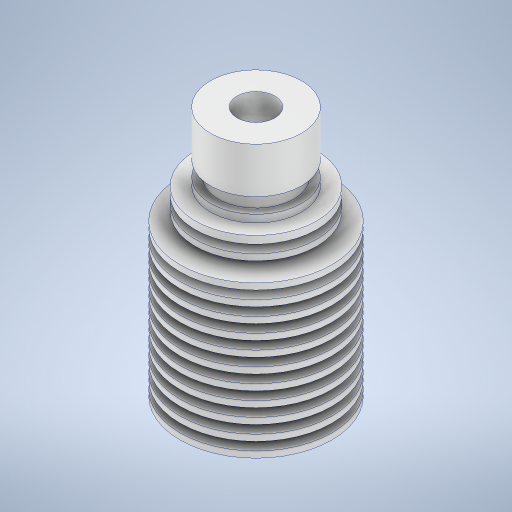
# Autodesk Inventor part: REVO-micro Heatsing body
Saved by Autodesk Inventor 2023.1 (Build 271208000, 208)
## iProperties
Created: 2022-11-20
Part Number: REVO-micro Heatsing body
Material: Aluminum 6061
Document SubType Name: Modeling
Designer: Frank
Density: 2.7 g/cm^3
Appearance: Aluminum - Flat
Mass: 12.3823 g
Surface Area: 79.4067 cm^2
Volume: 4.58604 cm^3
Author: Frank
Autodesk Inventor part; units mm, degrees
ref_plane "YZ Plane" through (0, 0, 0) normal (1, 0, 0) x (0, 1, 0)
ref_plane "XZ Plane" through (0, 0, 0) normal (0, 1, 0) x (-1, 0, 0)
ref_plane "XY Plane" through (0, 0, 0) normal (0, 0, 1) x (1, 0, 0)
sketch "Sketch1" plane through (0, 0, 0) normal (0, 0, 1) x (1, 0, 0)
  line L0 (0, 33) -> (0, -1)
  line L1 (0, -1) -> (3.75, -1) construction
  line L2 (3.75, -1) -> (3.75, 0)
  line L3 (3.75, 0) -> (10, 0)
  line L4 (10, 0) -> (10, 20)
  line L5 (10, 20) -> (8, 20)
  line L6 (8, 20) -> (8, 24)
  line L7 (8, 24) -> (6, 24)
  line L8 (6, 24) -> (6, 25)
  line L9 (6, 25) -> (5, 25)
  line L10 (5, 25) -> (5, 27)
  line L11 (5, 27) -> (6, 27)
  line L12 (6, 27) -> (6, 33)
  line L13 (6, 33) -> (0, 33)
  line L14 (10, 0) -> (0, 0) construction
  line L15 (6, 24) -> (6, 33) construction
  line L16 (2.5, 33) -> (2.5, 19)
  line L17 (2.5, 19) -> (1.55, 19)
  line L18 (1.55, 19) -> (1.55, 17)
  line L19 (1.55, 17) -> (2, 17)
  line L20 (10, 19.1818) -> (4.75, 19.1818)
  line L21 (4.75, 19.1818) -> (4.75, 18.0818)
  line L22 (4.75, 18.0818) -> (10, 18.0818)
  line L23 (10, 17.2636) -> (4.75, 17.2636)
  line L24 (4.75, 16.1636) -> (4.75, 17.2636)
  line L25 (4.75, 16.1636) -> (10, 16.1636)
  line L26 (10, 15.3455) -> (4.75, 15.3455)
  line L27 (4.75, 15.3455) -> (4.75, 14.2455)
  line L28 (4.75, 14.2455) -> (10, 14.2455)
  line L29 (10, 13.4273) -> (4.75, 13.4273)
  line L30 (4.75, 13.4273) -> (4.75, 12.3273)
  line L31 (4.75, 12.3273) -> (10, 12.3273)
  line L32 (10, 11.5091) -> (4.75, 11.5091)
  line L33 (4.75, 11.5091) -> (4.75, 10.4091)
  line L34 (4.75, 10.4091) -> (10, 10.4091)
  line L35 (10, 9.5909) -> (4.75, 9.5909)
  line L36 (4.75, 9.5909) -> (4.75, 8.4909)
  line L37 (4.75, 8.4909) -> (10, 8.4909)
  line L38 (10, 7.6727) -> (4.75, 7.6727)
  line L39 (4.75, 7.6727) -> (4.75, 6.5727)
  line L40 (4.75, 6.5727) -> (10, 6.5727)
  line L41 (10, 5.7545) -> (4.75, 5.7545)
  line L42 (4.75, 5.7545) -> (4.75, 4.6545)
  line L43 (4.75, 4.6545) -> (10, 4.6545)
  line L44 (4.75, 18.0818) -> (4.75, 17.2636) construction
  line L45 (4.75, 16.1636) -> (4.75, 15.3455) construction
  line L46 (4.75, 14.2455) -> (4.75, 13.4273) construction
  line L47 (4.75, 12.3273) -> (4.75, 11.5091) construction
  line L48 (4.75, 10.4091) -> (4.75, 9.5909) construction
  line L49 (4.75, 8.4909) -> (4.75, 7.6727) construction
  line L50 (4.75, 6.5727) -> (4.75, 5.7545) construction
  line L51 (10, 3.8364) -> (4.75, 3.8364)
  line L52 (4.75, 3.8364) -> (4.75, 2.7364)
  line L53 (4.75, 2.7364) -> (10, 2.7364)
  line L54 (10, 1.9182) -> (4.75, 1.9182)
  line L55 (4.75, 1.9182) -> (4.75, 0.8182)
  line L56 (4.75, 0.8182) -> (10, 0.8182)
  line L57 (4.75, 4.6545) -> (4.75, 3.8364) construction
  line L58 (4.75, 2.7364) -> (4.75, 1.9182) construction
  line L59 (4.75, 0) -> (4.75, 0.8182) construction
  line L60 (8, 20) -> (8, 19.1818) construction
  line L61 (8, 23) -> (4.75, 23)
  line L62 (4.75, 23) -> (4.75, 21.9)
  line L63 (4.75, 21.9) -> (8, 21.9)
  line L64 (8, 20) -> (4.75, 20)
  line L65 (8, 21.1) -> (4.75, 21.1)
  line L66 (4.75, 21.1) -> (4.75, 20)
  line L67 (3, -1) -> (3, 0)
  line L68 (3.75, -1) -> (3, -1)
  line L69 (2, 17) -> (2, 0)
  line L70 (3, 0) -> (2, 0)
  point P0 (5.5, 25)
  dimension "d2" = 12
  dimension "d3" = 20
  dimension "d4" = 7.5
  dimension "d5" = 20
  dimension "d6" = 16
  dimension "d7" = 10
  dimension "d11" = 6
  dimension "d12" = 8
  dimension "d13" = 33
  dimension "d14" = 5
  dimension "d16" = 3.1
  dimension "d17" = 17
  dimension "d18" = 14
  dimension "d19" = 9
  dimension "d21" = 1.1
  dimension "d25" = 9.5
  dimension "d26" = 1
  dimension "d27" = 0.8
  dimension "d28" = 1
  dimension "d29" = 6
  dimension "d30" = 4
  constraints: 140 end point, 23 perpendicular, 21 equal length, 20 horizontal, 19 point on line, 11 collinear, 8 vertical, 4 parallel, 1 midpoint, 23 other
  measures "d2" diameter of L12 L0
  measures "d4" diameter of L2 L0
  measures "d5" distance of L3.end L5.start
  measures "d6" diameter of L6 L0
  measures "d7" diameter of L10 L0
  measures "d11" distance between parallel lines of L13 L11
  measures "d12" distance between parallel lines of L13 L9
  measures "d13" distance between parallel lines of L13 L3
  measures "d14" diameter of L16 L0
  measures "d16" diameter of L18 L0
  measures "d17" distance between parallel lines of L14 L19
  measures "d18" distance between parallel lines of L13 L17
  measures "d19" distance between parallel lines of L13 L7
  measures "d21" distance between parallel lines of L22 L20
  measures "d25" diameter of L59.start L0
  measures "d26" distance between parallel lines of L7 L61
  measures "d27" distance between parallel lines of L65 L63
  measures "d28" distance of L1.end L2.end
  measures "d29" diameter of L67 L0
  measures "d30" diameter of L19.end L0
revolve "Revolution1" add sketch "Sketch1" angle 360 about axis through (0, 33, 0) along (0, -1, 0) contours L68 L67 L70 L69 L19 L18 L17 L16 L13 L12 L11 L10 L9 L8 L7 L6 L61 L62 L63 L65 L66 L64 L5 L4 L20 L21 L22 L23 L24 L25 L26 L27 L28 L29 L30 L31 L32 L33 L34 L35 L36 L37 L38 L39 L40 L41 L42 L43 L51 L52 L53 L54 L55 L56 L3 L2
body "Solid1"
